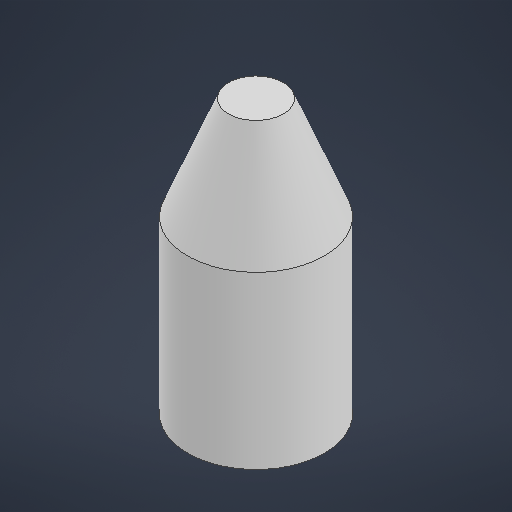
# Autodesk Inventor part: 针头
Saved by Autodesk Inventor 2025 (Build 290162000, 162)
## iProperties
Created: 2025-12-02
Part Number: 针头
Material: 常规
Document SubType Name: Modeling
Designer: XH
Density: 1 g/cm^3
Appearance: 默认
Author: XH
Autodesk Inventor part; units mm, degrees
ref_plane "YZ Plane" through (0, 0, 0) normal (1, 0, 0) x (0, 1, 0)
ref_plane "XZ Plane" through (0, 0, 0) normal (0, 1, 0) x (-1, 0, 0)
ref_plane "XY Plane" through (0, 0, 0) normal (0, 0, 1) x (1, 0, 0)
sketch "草图1" plane through (0, 0, 0) normal (0, 0, 1) x (1, 0, 0)
  line L0 (0, 0) -> (0, 5)
  line L1 (0, 5) -> (2, 0)
  line L2 (2, 0) -> (0, 0)
  line L3 (0, 3) -> (0.8, 3)
  dimension "d0" = 2
  dimension "d1" = 5
  dimension "d2" = 0.8
  constraints: 8 end point, 2 perpendicular, 2 point on line, 1 vertical
  measures "d0" distance of L1.end L0.start
  measures "d1" distance of L0.start L0.end
  measures "d2" distance of L3.start L3.end
revolve "旋转1" add sketch "草图1" angle 360 about axis through (0, 0, 0) along (0, 1, 0) contours L0 L3 L1 L2
sketch "草图2" plane through (0, 0, 0) normal (0, -1, 0) x (1, 0, 0)
  circle A0 centre (0, 0) radius 2 projected
extrude "拉伸1" add sketch "草图2" along normal blind 5
